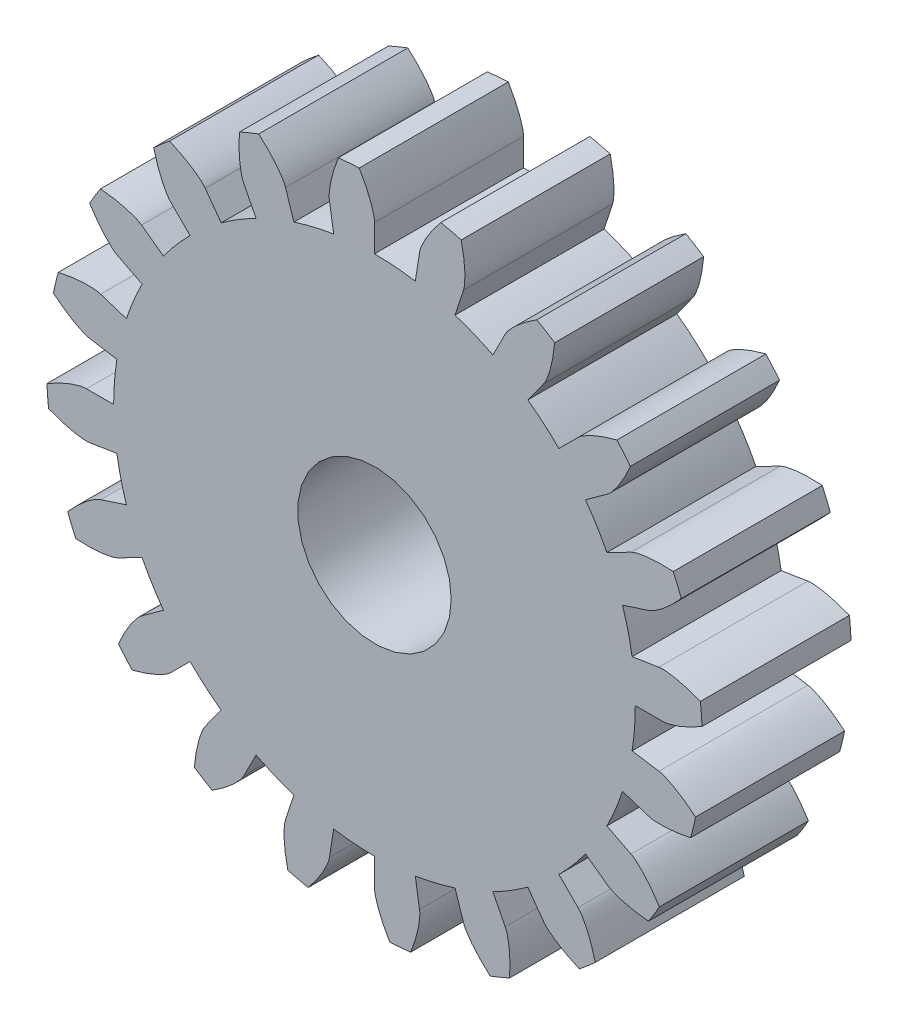
# Autodesk Inventor part: Gear_step1
Saved by Autodesk Inventor 2026.2 (Build 302298000, 298)
## iProperties
Created: 2025-12-18
Part Number: Gear_step1
Material: Generic
Document SubType Name: Modeling
Designer: Cobble
Density: 1 g/cm^3
Appearance: Default
Author: Cobble
Autodesk Inventor part; units mm, degrees
ref_plane "YZ Plane" through (0, 0, 0) normal (1, 0, 0) x (0, 1, 0)
ref_plane "XZ Plane" through (0, 0, 0) normal (0, 1, 0) x (-1, 0, 0)
ref_plane "XY Plane" through (0, 0, 0) normal (0, 0, 1) x (1, 0, 0)
sketch "Sketch1" plane through (0, 0, 0) normal (0, 0, 1) x (1, 0, 0)
  circle A0 centre (0, 0) radius 17.5
  circle A1 centre (0, 0) radius 22
  circle A2 centre (0, 0) radius 19.3185 construction
  line L0 (0, 0) -> (0, 30) construction
  line L1 (0, 0) -> (-9.2705, 28.5317) construction
  line L2 (0, 0) -> (-17.6336, 24.2705) construction
  line L3 (0, 0) -> (-24.2705, 17.6336) construction
  line L4 (0, 0) -> (-28.5317, 9.2705) construction
  line L5 (0, 0) -> (-30, 0) construction
  line L6 (0, 0) -> (-28.5317, -9.2705) construction
  line L7 (0, 0) -> (-24.2705, -17.6336) construction
  line L8 (0, 0) -> (-17.6336, -24.2705) construction
  line L9 (0, 0) -> (-9.2705, -28.5317) construction
  line L10 (0, 0) -> (0, -30) construction
  line L11 (0, 0) -> (9.2705, -28.5317) construction
  line L12 (0, 0) -> (17.6336, -24.2705) construction
  line L13 (0, 0) -> (24.2705, -17.6336) construction
  line L14 (0, 0) -> (28.5317, -9.2705) construction
  line L15 (0, 0) -> (30, 0) construction
  line L16 (0, 0) -> (28.5317, 9.2705) construction
  line L17 (0, 0) -> (24.2705, 17.6336) construction
  line L18 (0, 0) -> (17.6336, 24.2705) construction
  line L19 (0, 0) -> (9.2705, 28.5317) construction
  line L20 (-5.9697, 18.373) -> (-0.1988, 20.2481) construction
  line L21 (-11.3551, 15.629) -> (-1.537, 22.7623) construction
  line L22 (-15.629, 11.3551) -> (-4.9291, 26.0824) construction
  line L23 (-18.373, 5.9697) -> (-10.8726, 29.0536) construction
  spline S0 degree 4 poles (0, 19.3185) (0.0411, 20.4484) (-2.0761, 25.4109) (-6.0122, 27.0761) (-10.8726, 29.0536) knots 0 0 0 0 0 1 1 1 1 1
  spline S1 degree 4 poles (0, 19.3185) (0.0411, 20.4484) (-2.0761, 25.4109) (-6.0122, 27.0761) (-10.8726, 29.0536) knots 0 0 0 0 0 1 1 1 1 1 construction
  line L24 (0, 0) -> (-3.1287, 19.7538) construction
  line L25 (0, 0) -> (20, 0) construction
  line L26 (-1.0238, 21.9762) -> (0, 0) construction
  line L27 (-0.9557, 20.5152) -> (-0.2972, 20.5152) construction
  arc A3 (-0.1194, 19.9996) -> (-3.1287, 19.7538) centre (0, 0) ccw construction
  arc A4 (-5.5127, 19.2252) -> (6.1803, 19.0211) centre (0, 0) ccw construction
  line L28 (-5.8191, 18.4219) -> (0, 0) construction
  line L29 (0.2448, 18.7923) -> (0, 0) construction
  line L30 (-1.6287, 19.9336) -> (0, 0)
  line L31 (0, 0) -> (4.3949, 27.7482) construction
  line L32 (0, 0) -> (28.0941, 0) construction
  line L33 (0, 0) -> (-4.3949, 27.7482) construction
  line L34 (0, 0) -> (-12.7545, 25.032) construction
  line L35 (0, 0) -> (-19.8655, 19.8655) construction
  line L36 (0, 0) -> (-25.032, 12.7545) construction
  line L37 (0, 0) -> (-27.7482, 4.3949) construction
  line L38 (0, 0) -> (-27.7482, -4.3949) construction
  line L39 (0, 0) -> (-25.032, -12.7545) construction
  line L40 (0, 0) -> (-19.8655, -19.8655) construction
  line L41 (0, 0) -> (-12.7545, -25.032) construction
  line L42 (0, 0) -> (-4.3949, -27.7482) construction
  line L43 (0, 0) -> (4.3949, -27.7482) construction
  line L44 (0, 0) -> (12.7545, -25.032) construction
  line L45 (0, 0) -> (19.8655, -19.8655) construction
  line L46 (0, 0) -> (25.032, -12.7545) construction
  line L47 (0, 0) -> (27.7482, -4.3949) construction
  line L48 (0, 0) -> (27.7482, 4.3949) construction
  line L49 (0, 0) -> (25.032, 12.7545) construction
  line L50 (0, 0) -> (19.8655, 19.8655) construction
  line L51 (0, 0) -> (12.7545, 25.032) construction
  line L52 (3.0221, 19.0807) -> (-2.9712, 20.0299) construction
  line L53 (8.7704, 17.2129) -> (-2.0427, 22.7225) construction
  line L54 (13.6603, 13.6603) -> (0.7882, 26.5323) construction
  line L55 (17.2129, 8.7704) -> (6.1938, 30.3967) construction
  spline S2 degree 4 poles (-3.0221, 19.0807) (-3.2394, 20.1903) (-1.9246, 25.4228) (1.7025, 27.6832) (6.1938, 30.3967) knots 0 0 0 0 0 1 1 1 1 1
  line L56 (-3.0221, 19.0807) -> (0, 0)
  line L57 (0, 19.3185) -> (0, 0)
  line L58 (0, 0) -> (-9.0798, 17.8201) construction
  spline S3 degree 4 poles (-5.9697, 18.373) (-6.2798, 19.4603) (-9.8269, 23.5257) (-14.0849, 23.893) (-19.3185, 24.2718) knots 0 0 0 0 0 1 1 1 1 1
  spline S4 degree 4 poles (-8.7704, 17.2129) (-9.32, 18.201) (-9.6865, 23.5838) (-6.9354, 26.8544) (-3.5025, 30.823) knots 0 0 0 0 0 1 1 1 1 1
  line L59 (0, 0) -> (-9.2705, 28.5317) construction
  line L60 (-8.7704, 17.2129) -> (0, 0)
  line L61 (-5.9697, 18.373) -> (0, 0)
  line L62 (0, 0) -> (-14.1421, 14.1421) construction
  spline S5 degree 4 poles (-11.3551, 15.629) (-11.986, 16.5673) (-16.6157, 19.3376) (-20.7789, 18.3711) (-25.8734, 17.1141) knots 0 0 0 0 0 1 1 1 1 1
  spline S6 degree 4 poles (-13.6603, 13.6603) (-14.4883, 14.4302) (-16.5002, 19.4362) (-14.8944, 23.3969) (-12.8559, 28.2321) knots 0 0 0 0 0 1 1 1 1 1
  line L63 (0, 0) -> (-17.6336, 24.2705) construction
  line L64 (-13.6603, 13.6603) -> (0, 0)
  line L65 (-11.3551, 15.629) -> (0, 0)
  line L66 (0, 0) -> (-17.8201, 9.0798) construction
  spline S7 degree 4 poles (-15.629, 11.3551) (-16.519, 12.0526) (-21.7781, 13.2566) (-25.4389, 11.051) (-29.8956, 8.2811) knots 0 0 0 0 0 1 1 1 1 1
  spline S8 degree 4 poles (-17.2129, 8.7704) (-18.2384, 9.2468) (-21.6988, 13.3861) (-21.3955, 17.6492) (-20.9509, 22.8776) knots 0 0 0 0 0 1 1 1 1 1
  line L67 (0, 0) -> (-24.2705, 17.6336) construction
  line L68 (-17.2129, 8.7704) -> (0, 0)
  line L69 (-15.629, 11.3551) -> (0, 0)
  line L70 (0, 0) -> (-19.7538, 3.1287) construction
  spline S9 degree 4 poles (-18.373, 5.9697) (-19.4349, 6.358) (-24.8088, 5.878) (-27.6087, 2.649) (-30.9914, -1.3624) knots 0 0 0 0 0 1 1 1 1 1
  spline S10 degree 4 poles (-19.0807, 3.0221) (-20.2031, 3.1582) (-24.7733, 6.0256) (-25.8022, 10.1738) (-26.995, 15.2837) knots 0 0 0 0 0 1 1 1 1 1
  line L71 (0, 0) -> (-28.5317, 9.2705) construction
  line L72 (-19.0807, 3.0221) -> (0, 0)
  line L73 (-18.373, 5.9697) -> (0, 0)
  line L74 (0, 0) -> (-19.7538, -3.1287) construction
  spline S11 degree 4 poles (-19.3185, 0) (-20.4484, 0.0411) (-25.4109, -2.0761) (-27.0761, -6.0122) (-29.0536, -10.8726) knots 0 0 0 0 0 1 1 1 1 1
  spline S12 degree 4 poles (-19.0807, -3.0221) (-20.1903, -3.2394) (-25.4228, -1.9246) (-27.6832, 1.7025) (-30.3967, 6.1938) knots 0 0 0 0 0 1 1 1 1 1
  line L75 (0, 0) -> (-30, 0) construction
  line L76 (-19.0807, -3.0221) -> (0, 0)
  line L77 (-19.3185, 0) -> (0, 0)
  line L78 (0, 0) -> (-17.8201, -9.0798) construction
  spline S13 degree 4 poles (-18.373, -5.9697) (-19.4603, -6.2798) (-23.5257, -9.8269) (-23.893, -14.0849) (-24.2718, -19.3185) knots 0 0 0 0 0 1 1 1 1 1
  spline S14 degree 4 poles (-17.2129, -8.7704) (-18.201, -9.32) (-23.5838, -9.6865) (-26.8544, -6.9354) (-30.823, -3.5025) knots 0 0 0 0 0 1 1 1 1 1
  line L79 (0, 0) -> (-28.5317, -9.2705) construction
  line L80 (-17.2129, -8.7704) -> (0, 0)
  line L81 (-18.373, -5.9697) -> (0, 0)
  line L82 (0, 0) -> (-14.1421, -14.1421) construction
  spline S15 degree 4 poles (-15.629, -11.3551) (-16.5673, -11.986) (-19.3376, -16.6157) (-18.3711, -20.7789) (-17.1141, -25.8734) knots 0 0 0 0 0 1 1 1 1 1
  spline S16 degree 4 poles (-13.6603, -13.6603) (-14.4302, -14.4883) (-19.4362, -16.5002) (-23.3969, -14.8944) (-28.2321, -12.8559) knots 0 0 0 0 0 1 1 1 1 1
  line L83 (0, 0) -> (-24.2705, -17.6336) construction
  line L84 (-13.6603, -13.6603) -> (0, 0)
  line L85 (-15.629, -11.3551) -> (0, 0)
  line L86 (0, 0) -> (-9.0798, -17.8201) construction
  spline S17 degree 4 poles (-11.3551, -15.629) (-12.0526, -16.519) (-13.2566, -21.7781) (-11.051, -25.4389) (-8.2811, -29.8956) knots 0 0 0 0 0 1 1 1 1 1
  spline S18 degree 4 poles (-8.7704, -17.2129) (-9.2468, -18.2384) (-13.3861, -21.6988) (-17.6492, -21.3955) (-22.8776, -20.9509) knots 0 0 0 0 0 1 1 1 1 1
  line L87 (0, 0) -> (-17.6336, -24.2705) construction
  line L88 (-8.7704, -17.2129) -> (0, 0)
  line L89 (-11.3551, -15.629) -> (0, 0)
  line L90 (0, 0) -> (-3.1287, -19.7538) construction
  spline S19 degree 4 poles (-5.9697, -18.373) (-6.358, -19.4349) (-5.878, -24.8088) (-2.649, -27.6087) (1.3624, -30.9914) knots 0 0 0 0 0 1 1 1 1 1
  spline S20 degree 4 poles (-3.0221, -19.0807) (-3.1582, -20.2031) (-6.0256, -24.7733) (-10.1738, -25.8022) (-15.2837, -26.995) knots 0 0 0 0 0 1 1 1 1 1
  line L91 (0, 0) -> (-9.2705, -28.5317) construction
  line L92 (-3.0221, -19.0807) -> (0, 0)
  line L93 (-5.9697, -18.373) -> (0, 0)
  line L94 (0, 0) -> (3.1287, -19.7538) construction
  spline S21 degree 4 poles (0, -19.3185) (-0.0411, -20.4484) (2.0761, -25.4109) (6.0122, -27.0761) (10.8726, -29.0536) knots 0 0 0 0 0 1 1 1 1 1
  spline S22 degree 4 poles (3.0221, -19.0807) (3.2394, -20.1903) (1.9246, -25.4228) (-1.7025, -27.6832) (-6.1938, -30.3967) knots 0 0 0 0 0 1 1 1 1 1
  line L95 (0, 0) -> (0, -30) construction
  line L96 (3.0221, -19.0807) -> (0, 0)
  line L97 (0, -19.3185) -> (0, 0)
  line L98 (0, 0) -> (9.0798, -17.8201) construction
  spline S23 degree 4 poles (5.9697, -18.373) (6.2798, -19.4603) (9.8269, -23.5257) (14.0849, -23.893) (19.3185, -24.2718) knots 0 0 0 0 0 1 1 1 1 1
  spline S24 degree 4 poles (8.7704, -17.2129) (9.32, -18.201) (9.6865, -23.5838) (6.9354, -26.8544) (3.5025, -30.823) knots 0 0 0 0 0 1 1 1 1 1
  line L99 (0, 0) -> (9.2705, -28.5317) construction
  line L100 (8.7704, -17.2129) -> (0, 0)
  line L101 (5.9697, -18.373) -> (0, 0)
  line L102 (0, 0) -> (14.1421, -14.1421) construction
  spline S25 degree 4 poles (11.3551, -15.629) (11.986, -16.5673) (16.6157, -19.3376) (20.7789, -18.3711) (25.8734, -17.1141) knots 0 0 0 0 0 1 1 1 1 1
  spline S26 degree 4 poles (13.6603, -13.6603) (14.4883, -14.4302) (16.5002, -19.4362) (14.8944, -23.3969) (12.8559, -28.2321) knots 0 0 0 0 0 1 1 1 1 1
  line L103 (0, 0) -> (17.6336, -24.2705) construction
  line L104 (13.6603, -13.6603) -> (0, 0)
  line L105 (11.3551, -15.629) -> (0, 0)
  line L106 (0, 0) -> (17.8201, -9.0798) construction
  spline S27 degree 4 poles (15.629, -11.3551) (16.519, -12.0526) (21.7781, -13.2566) (25.4389, -11.051) (29.8956, -8.2811) knots 0 0 0 0 0 1 1 1 1 1
  spline S28 degree 4 poles (17.2129, -8.7704) (18.2384, -9.2468) (21.6988, -13.3861) (21.3955, -17.6492) (20.9509, -22.8776) knots 0 0 0 0 0 1 1 1 1 1
  line L107 (0, 0) -> (24.2705, -17.6336) construction
  line L108 (17.2129, -8.7704) -> (0, 0)
  line L109 (15.629, -11.3551) -> (0, 0)
  line L110 (0, 0) -> (19.7538, -3.1287) construction
  spline S29 degree 4 poles (18.373, -5.9697) (19.4349, -6.358) (24.8088, -5.878) (27.6087, -2.649) (30.9914, 1.3624) knots 0 0 0 0 0 1 1 1 1 1
  spline S30 degree 4 poles (19.0807, -3.0221) (20.2031, -3.1582) (24.7733, -6.0256) (25.8022, -10.1738) (26.995, -15.2837) knots 0 0 0 0 0 1 1 1 1 1
  line L111 (0, 0) -> (28.5317, -9.2705) construction
  line L112 (19.0807, -3.0221) -> (0, 0)
  line L113 (18.373, -5.9697) -> (0, 0)
  line L114 (0, 0) -> (19.7538, 3.1287) construction
  spline S31 degree 4 poles (19.3185, 0) (20.4484, -0.0411) (25.4109, 2.0761) (27.0761, 6.0122) (29.0536, 10.8726) knots 0 0 0 0 0 1 1 1 1 1
  spline S32 degree 4 poles (19.0807, 3.0221) (20.1903, 3.2394) (25.4228, 1.9246) (27.6832, -1.7025) (30.3967, -6.1938) knots 0 0 0 0 0 1 1 1 1 1
  line L115 (0, 0) -> (30, 0) construction
  line L116 (19.0807, 3.0221) -> (0, 0)
  line L117 (19.3185, 0) -> (0, 0)
  line L118 (0, 0) -> (17.8201, 9.0798) construction
  spline S33 degree 4 poles (18.373, 5.9697) (19.4603, 6.2798) (23.5257, 9.8269) (23.893, 14.0849) (24.2718, 19.3185) knots 0 0 0 0 0 1 1 1 1 1
  spline S34 degree 4 poles (17.2129, 8.7704) (18.201, 9.32) (23.5838, 9.6865) (26.8544, 6.9354) (30.823, 3.5025) knots 0 0 0 0 0 1 1 1 1 1
  line L119 (0, 0) -> (28.5317, 9.2705) construction
  line L120 (17.2129, 8.7704) -> (0, 0)
  line L121 (18.373, 5.9697) -> (0, 0)
  line L122 (0, 0) -> (14.1421, 14.1421) construction
  spline S35 degree 4 poles (15.629, 11.3551) (16.5673, 11.986) (19.3376, 16.6157) (18.3711, 20.7789) (17.1141, 25.8734) knots 0 0 0 0 0 1 1 1 1 1
  spline S36 degree 4 poles (13.6603, 13.6603) (14.4302, 14.4883) (19.4362, 16.5002) (23.3969, 14.8944) (28.2321, 12.8559) knots 0 0 0 0 0 1 1 1 1 1
  line L123 (0, 0) -> (24.2705, 17.6336) construction
  line L124 (13.6603, 13.6603) -> (0, 0)
  line L125 (15.629, 11.3551) -> (0, 0)
  line L126 (0, 0) -> (9.0798, 17.8201) construction
  spline S37 degree 4 poles (11.3551, 15.629) (12.0526, 16.519) (13.2566, 21.7781) (11.051, 25.4389) (8.2811, 29.8956) knots 0 0 0 0 0 1 1 1 1 1
  spline S38 degree 4 poles (8.7704, 17.2129) (9.2468, 18.2384) (13.3861, 21.6988) (17.6492, 21.3955) (22.8776, 20.9509) knots 0 0 0 0 0 1 1 1 1 1
  line L127 (0, 0) -> (17.6336, 24.2705) construction
  line L128 (8.7704, 17.2129) -> (0, 0)
  line L129 (11.3551, 15.629) -> (0, 0)
  line L130 (0, 0) -> (3.1287, 19.7538) construction
  spline S39 degree 4 poles (5.9697, 18.373) (6.358, 19.4349) (5.878, 24.8088) (2.649, 27.6087) (-1.3624, 30.9914) knots 0 0 0 0 0 1 1 1 1 1
  spline S40 degree 4 poles (3.0221, 19.0807) (3.1582, 20.2031) (6.0256, 24.7733) (10.1738, 25.8022) (15.2837, 26.995) knots 0 0 0 0 0 1 1 1 1 1
  line L131 (0, 0) -> (9.2705, 28.5317) construction
  line L132 (3.0221, 19.0807) -> (0, 0)
  line L133 (5.9697, 18.373) -> (0, 0)
  circle A5 centre (0, 0) radius 20
  point P0 (0.1192, 17.4996)
  point P1 (-6.4461, 19.1957)
  point P2 (-8.4957, 21.1733)
  point P3 (-12.7477, 23.2826)
  point P4 (-9.0153, 18.1314)
  point P5 (-8.9644, 20.9791)
  point P6 (-7.4493, 25.4773)
  point P7 (-12.0624, 16.2642)
  point P8 (-14.6228, 17.5117)
  point P9 (-19.3185, 18.2038)
  point P10 (-14.177, 14.4581)
  point P11 (-15.0086, 17.1822)
  point P12 (-14.9576, 21.9284)
  point P13 (-16.4979, 11.7407)
  point P14 (-19.3185, 12.1359)
  point P15 (-23.9983, 11.3431)
  point P16 (-17.9509, 9.3696)
  point P17 (-19.5836, 11.7033)
  point P18 (-21.0018, 16.233)
  point P19 (-19.3185, 6.0679)
  point P20 (-22.1232, 5.5722)
  point P21 (-26.329, 3.3721)
  point P22 (-19.9677, 3.3638)
  point P23 (-22.2416, 5.0789)
  point P24 (-24.9902, 8.9486)
  point P25 (-20.2481, -0.1988)
  point P26 (-22.7623, -1.537)
  point P27 (-26.0824, -4.9291)
  point P28 (-20.0299, -2.9712)
  point P29 (-22.7225, -2.0427)
  point P30 (-26.5323, 0.7882)
  point P31 (-19.1957, -6.4461)
  point P32 (-21.1733, -8.4957)
  point P33 (-23.2826, -12.7477)
  point P34 (-18.1314, -9.0153)
  point P35 (-20.9791, -8.9644)
  point P36 (-25.4773, -7.4493)
  point P37 (-16.2642, -12.0624)
  point P38 (-17.5117, -14.6228)
  point P39 (-18.2038, -19.3185)
  point P40 (-14.4581, -14.177)
  point P41 (-17.1822, -15.0086)
  point P42 (-21.9284, -14.9576)
  point P43 (-11.7407, -16.4979)
  point P44 (-12.1359, -19.3185)
  point P45 (-11.3431, -23.9983)
  point P46 (-9.3696, -17.9509)
  point P47 (-11.7033, -19.5836)
  point P48 (-16.233, -21.0018)
  point P49 (-6.0679, -19.3185)
  point P50 (-5.5722, -22.1232)
  point P51 (-3.3721, -26.329)
  point P52 (-3.3638, -19.9677)
  point P53 (-5.0789, -22.2416)
  point P54 (-8.9486, -24.9902)
  point P55 (0.1988, -20.2481)
  point P56 (1.537, -22.7623)
  point P57 (4.9291, -26.0824)
  point P58 (2.9712, -20.0299)
  point P59 (2.0427, -22.7225)
  point P60 (-0.7882, -26.5323)
  point P61 (6.4461, -19.1957)
  point P62 (8.4957, -21.1733)
  point P63 (12.7477, -23.2826)
  point P64 (9.0153, -18.1314)
  point P65 (8.9644, -20.9791)
  point P66 (7.4493, -25.4773)
  point P67 (12.0624, -16.2642)
  point P68 (14.6228, -17.5117)
  point P69 (19.3185, -18.2038)
  point P70 (14.177, -14.4581)
  point P71 (15.0086, -17.1822)
  point P72 (14.9576, -21.9284)
  point P73 (16.4979, -11.7407)
  point P74 (19.3185, -12.1359)
  point P75 (23.9983, -11.3431)
  point P76 (17.9509, -9.3696)
  point P77 (19.5836, -11.7033)
  point P78 (21.0018, -16.233)
  point P79 (19.3185, -6.0679)
  point P80 (22.1232, -5.5722)
  point P81 (26.329, -3.3721)
  point P82 (19.9677, -3.3638)
  point P83 (22.2416, -5.0789)
  point P84 (24.9902, -8.9486)
  point P85 (20.2481, 0.1988)
  point P86 (22.7623, 1.537)
  point P87 (26.0824, 4.9291)
  point P88 (20.0299, 2.9712)
  point P89 (22.7225, 2.0427)
  point P90 (26.5323, -0.7882)
  point P91 (19.1957, 6.4461)
  point P92 (21.1733, 8.4957)
  point P93 (23.2826, 12.7477)
  point P94 (18.1314, 9.0153)
  point P95 (20.9791, 8.9644)
  point P96 (25.4773, 7.4493)
  point P97 (16.2642, 12.0624)
  point P98 (17.5117, 14.6228)
  point P99 (18.2038, 19.3185)
  point P100 (14.4581, 14.177)
  point P101 (17.1822, 15.0086)
  point P102 (21.9284, 14.9576)
  point P103 (11.7407, 16.4979)
  point P104 (12.1359, 19.3185)
  point P105 (11.3431, 23.9983)
  point P106 (9.3696, 17.9509)
  point P107 (11.7033, 19.5836)
  point P108 (16.233, 21.0018)
  point P109 (6.0679, 19.3185)
  point P110 (5.5722, 22.1232)
  point P111 (3.3721, 26.329)
  point P112 (3.3638, 19.9677)
  point P113 (5.0789, 22.2416)
  point P114 (8.9486, 24.9902)
  point P115 (-2.7376, 17.2845)
  point P116 (-5.4078, 16.6435)
  point P117 (-7.7647, 20.5842)
  point P118 (-9.0648, 20.0457)
  point P119 (-8.7704, 17.2129)
  point P120 (-7.9448, 15.5926)
  point P121 (-10.2862, 14.1578)
  point P122 (-13.7455, 17.1773)
  point P123 (-14.8156, 16.2634)
  point P124 (-13.6603, 13.6603)
  point P125 (-12.3744, 12.3744)
  point P126 (-14.1578, 10.2862)
  point P127 (-18.3809, 12.089)
  point P128 (-19.1161, 10.8892)
  point P129 (-15.5926, 7.9448)
  point P130 (-16.6435, 5.4078)
  point P131 (-21.2169, 5.8173)
  point P132 (-21.5454, 4.449)
  point P133 (-17.2845, 2.7376)
  point P134 (-17.5, 0)
  point P135 (-21.9762, -1.0238)
  point P136 (-21.8658, -2.4266)
  point P137 (-19.0807, -3.0221)
  point P138 (-17.2845, -2.7376)
  point P139 (-16.6435, -5.4078)
  point P140 (-20.5842, -7.7647)
  point P141 (-20.0457, -9.0648)
  point P142 (-17.2129, -8.7704)
  point P143 (-15.5926, -7.9448)
  point P144 (-14.1578, -10.2862)
  point P145 (-17.1773, -13.7455)
  point P146 (-16.2634, -14.8156)
  point P147 (-13.6603, -13.6603)
  point P148 (-12.3744, -12.3744)
  point P149 (-10.2862, -14.1578)
  point P150 (-12.089, -18.3809)
  point P151 (-10.8892, -19.1161)
  point P152 (-8.7704, -17.2129)
  point P153 (-7.9448, -15.5926)
  point P154 (-5.4078, -16.6435)
  point P155 (-5.8173, -21.2169)
  point P156 (-4.449, -21.5454)
  point P157 (-3.0221, -19.0807)
  point P158 (-2.7376, -17.2845)
  point P159 (0, -17.5)
  point P160 (1.0238, -21.9762)
  point P161 (2.4266, -21.8658)
  point P162 (3.0221, -19.0807)
  point P163 (2.7376, -17.2845)
  point P164 (5.4078, -16.6435)
  point P165 (7.7647, -20.5842)
  point P166 (9.0648, -20.0457)
  point P167 (7.9448, -15.5926)
  point P168 (10.2862, -14.1578)
  point P169 (13.7455, -17.1773)
  point P170 (14.8156, -16.2634)
  point P171 (12.3744, -12.3744)
  point P172 (14.1578, -10.2862)
  point P173 (18.3809, -12.089)
  point P174 (19.1161, -10.8892)
  point P175 (17.2129, -8.7704)
  point P176 (15.5926, -7.9448)
  point P177 (16.6435, -5.4078)
  point P178 (21.2169, -5.8173)
  point P179 (21.5454, -4.449)
  point P180 (19.0807, -3.0221)
  point P181 (17.2845, -2.7376)
  point P182 (17.5, 0)
  point P183 (21.9762, 1.0238)
  point P184 (21.8658, 2.4266)
  point P185 (19.0807, 3.0221)
  point P186 (17.2845, 2.7376)
  point P187 (16.6435, 5.4078)
  point P188 (20.5842, 7.7647)
  point P189 (20.0457, 9.0648)
  point P190 (15.5926, 7.9448)
  point P191 (14.1578, 10.2862)
  point P192 (17.1773, 13.7455)
  point P193 (16.2634, 14.8156)
  point P194 (13.6603, 13.6603)
  point P195 (12.3744, 12.3744)
  point P196 (10.2862, 14.1578)
  point P197 (12.089, 18.3809)
  point P198 (10.8892, 19.1161)
  point P199 (8.7704, 17.2129)
  dimension "d1" = 35
  dimension "d2" = 44
  dimension "d3" = 38.637
  dimension "d4" = 30
  dimension "d7" = 360
  dimension "d9" = 6.0679
  dimension "d10" = 12.1359
  dimension "d11" = 18.2038
  dimension "d12" = 24.2718
  dimension "d14" = 99
  dimension "d24" = 81
  dimension "d27" = 360
  dimension "d29" = 6.0679
  dimension "d30" = 12.1359
  dimension "d31" = 18.2038
  dimension "d32" = 24.2718
  dimension "d35" = 360
  dimension "d37" = 40
  constraints: 268 end point, 32 point on line, 7 perpendicular, 5 coincident, 5 point on circle, 4 horizontal, 3 centre point, 2 collinear, 2 equal length, 1 vertical, 798 other
  measures "d4" distance of L0.start L0.end
  measures "d9" distance of L20.start L20.end
  measures "d10" distance of L21.start L21.end
  measures "d11" distance of L22.start L22.end
  measures "d12" distance of L23.start L23.end
  measures "d14" angle of L25 L24
  measures "d24" angle of L32 L31
  measures "d29" distance of L52.start L52.end
  measures "d30" distance of L53.start L53.end
  measures "d31" distance of L54.start L54.end
  measures "d32" distance of L55.start L55.end
  measures "d37" diameter of A5
extrude "Extrusion1" add sketch "Sketch1" along normal blind 10 contours L117 L116 A0 | A0 L116 S32 A5 S31 L117 | A0 L112 L117 | L116 L121 A0 | L112 S30 A5 S29 L113 A0 | A0 L113 L112 | L56 A0 L30 | L61 A0 L56 | L30 A0 L57 | L65 A0 L60 | L60 A0 L61 | L69 A0 L64 | L64 A0 L65 | L73 A0 L68 | L68 A0 L69 | L77 A0 L72 | L72 A0 L73 | L81 A0 L76 | L76 A0 L77 | L85 A0 L80 | L80 A0 L81 | L89 A0 L84 | L84 A0 L85 | L93 A0 L88 | L88 A0 L89 | L97 A0 L92 | L92 A0 L93 | L101 A0 L96 | L96 A0 L97 | L105 A0 L100 | L100 A0 L101 | L109 A0 L104 | L104 A0 L105 | L113 A0 L108 | L108 A0 L109 | L125 A0 L120 | L120 A0 L121 | L129 A0 L124 | L124 A0 L125 | L133 A0 L128 | L128 A0 L129 | L57 A0 L132 | L132 A0 L133 | A0 L120 S34 A5 S33 L121 | A5 S32 A1 S31 | L30 A5 S0 L57 A0 | A0 L56 S2 A5 L30 | L60 S4 A5 S3 L61 A0 | L64 S6 A5 S5 L65 A0 | L68 S8 A5 S7 L69 A0 | L72 S10 A5 S9 L73 A0 | L76 S12 A5 S11 L77 A0 | L80 S14 A5 S13 L81 A0 | L84 S16 A5 S15 L85 A0 | L88 S18 A5 S17 L89 A0 | L92 S20 A5 S19 L93 A0 | L96 S22 A5 S21 L97 A0 | L100 S24 A5 S23 L101 A0 | L104 S26 A5 S25 L105 A0 | L108 S28 A5 S27 L109 A0 | L124 S36 A5 S35 L125 A0 | L128 S38 A5 S37 L129 A0 | L132 S40 A5 S39 L133 A0 | S30 A1 S29 A5 | A5 S2 A1 S0 | A5 S34 A1 S33 | S4 A1 S3 A5 | S6 A1 S5 A5 | S8 A1 S7 A5 | S10 A1 S9 A5 | S12 A1 S11 A5 | S14 A1 S13 A5 | S16 A1 S15 A5 | S18 A1 S17 A5 | S20 A1 S19 A5 | S22 A1 S21 A5 | S24 A1 S23 A5 | S26 A1 S25 A5 | S28 A1 S27 A5 | S36 A1 S35 A5 | S38 A1 S37 A5 | S40 A1 S39 A5
sketch "Sketch2" plane through (0, 0, 10) normal (0, 0, 1) x (1, 0, 0)
  circle A0 centre (0, 0) radius 5.15
  dimension "d21" = 10.3
  constraints: 1 centre point, 1 coincident
  measures "d21" diameter of A0
extrude "Extrusion2" cut sketch "Sketch2" against normal blind 10
equation "\"d3\" = 0.965926 * d37"
equation "\"d9\" = 0.15705 * d3"
equation "\"d10\" = 2 * d9"
equation "\"d11\" = 3 * d9"
equation "\"d12\" = 4 * d9"
equation "\"d29\" = d9"
equation "\"d30\" = d10"
equation "\"d31\" = d11"
equation "\"d32\" = d12"
body "Solid1"
